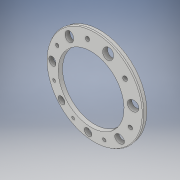
# Autodesk Inventor part: Component 10(Assembly Ring)
Saved by Autodesk Inventor 2018 (Build 220112000, 112)
## iProperties
Created: 2023-03-14
Part Number: Component 10(Assembly Ring)
Material: Generic
Document SubType Name: Modeling
Designer: Habib Mohamed
Density: 1 g/cm^3
Appearance: Default
Author: Habib Mohamed
Autodesk Inventor part; units mm, degrees
ref_plane "YZ Plane" through (0, 0, 0) normal (1, 0, 0) x (0, 1, 0)
ref_plane "XZ Plane" through (0, 0, 0) normal (0, 1, 0) x (-1, 0, 0)
ref_plane "XY Plane" through (0, 0, 0) normal (0, 0, 1) x (1, 0, 0)
sketch "Sketch1" plane through (0, 0, 0) normal (0, 0, 1) x (1, 0, 0)
  circle A0 centre (0, 0) radius 45
  circle A1 centre (0, 0) radius 65
  circle A2 centre (0, 0) radius 55 construction
  circle A3 centre (0, -55) radius 6
  circle A4 centre (0, 55) radius 2.5
  line L0 (0, 0) -> (0, 34.6858) construction
  circle A5 centre (-43.0007, 34.2919) radius 2.5
  circle A6 centre (43.0007, -34.2919) radius 6
  circle A7 centre (-53.621, -12.2387) radius 2.5
  circle A8 centre (53.621, 12.2387) radius 6
  circle A9 centre (-23.8636, -49.5533) radius 2.5
  circle A10 centre (23.8636, 49.5533) radius 6
  circle A11 centre (23.8636, -49.5533) radius 2.5
  circle A12 centre (-23.8636, 49.5533) radius 6
  circle A13 centre (53.621, -12.2387) radius 2.5
  circle A14 centre (-53.621, 12.2387) radius 6
  circle A15 centre (43.0007, 34.2919) radius 2.5
  circle A16 centre (-43.0007, -34.2919) radius 6
  point P0 (0, 17.3429)
  dimension "d0" = 90
  dimension "d1" = 130
  dimension "d2" = 110
  dimension "d3" = 12
  dimension "d4" = 5
  dimension "d7" = 360
  constraints: 17 centre point, 3 coincident, 2 end point, 2 point on circle, 1 midpoint, 1 point on line, 1 vertical, 1 vertical alignment, 29 other
  measures "d0" diameter of A0
  measures "d1" diameter of A1
  measures "d2" diameter of A2
  measures "d3" diameter of A3
  measures "d4" diameter of A4
extrude "Extrusion1" add sketch "Sketch1" along normal blind 6
fillet "Fillet1" radius 1 2 edges at (-65, 0, 6) (-65, 0, 0)
body "Solid1"
